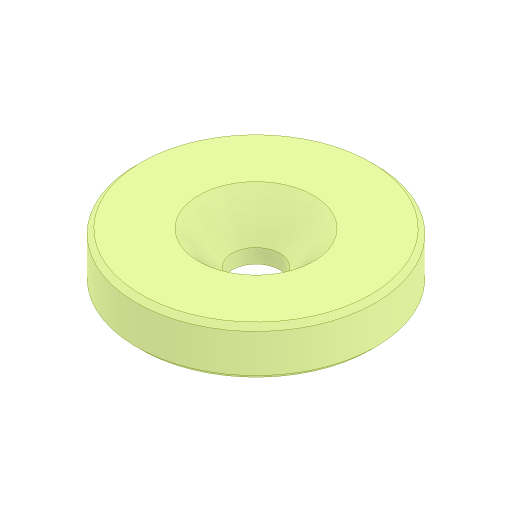
# Autodesk Inventor part: Magnet
Saved by Autodesk Inventor 2024.3 (Build 283343000, 343)
## iProperties
Created: 2025-05-16
Part Number: Magnet
Material: Generisch
Document SubType Name: Modeling
Designer: Demir
Density: 1 g/cm^3
Appearance: Zinkchromat 2
Author: Demir
Autodesk Inventor part; units mm, degrees
ref_plane "YZ Plane" through (0, 0, 0) normal (1, 0, 0) x (0, 1, 0)
ref_plane "XZ Plane" through (0, 0, 0) normal (0, 1, 0) x (-1, 0, 0)
ref_plane "XY Plane" through (0, 0, 0) normal (0, 0, 1) x (1, 0, 0)
sketch "Skizze1" plane through (0, 0, 0) normal (0, 0, 1) x (1, 0, 0)
  circle A0 centre (0, 0) radius 12.5
  dimension "d0" = 25
  constraints: 1 centre point, 1 coincident
  measures "d0" diameter of A0
extrude "Extrusion1" add sketch "Skizze1" along normal blind 5
chamfer "Fasen1" distance 0.5 angle 45 2 edges at (-12.5, 0, 0) (-12.5, 0, 5)
sketch "Skizze2" plane through (0, 0, 5) normal (0, 0, 1) x (1, 0, 0)
  circle A0 centre (0, 0) radius 12 projected
  constraints: 1 coincident
hole "Bohrung1" at (0, 0, 5) direction (0, 0, -1) diameter 5 end through all countersink diameter 12 countersink angle 90
